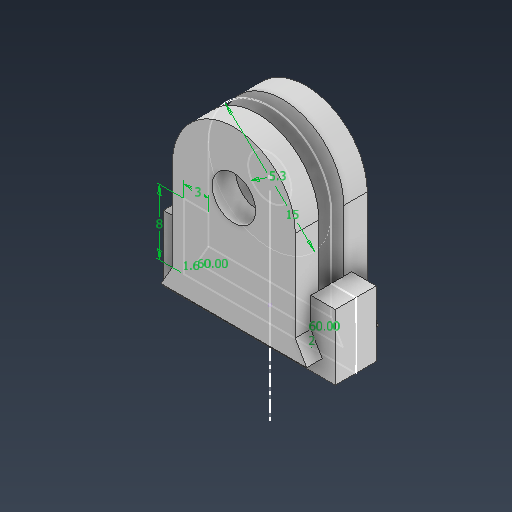
# Autodesk Inventor part: base
Saved by Autodesk Inventor 2025.3 (Build 293356000, 356)
## iProperties
Created: 2025-11-24
Part Number: base
Material: 一般
Document SubType Name: Modeling
Designer: 陳泓任
Density: 1 g/cm^3
Appearance: 預設
Author: 陳泓任
Autodesk Inventor part; units mm, degrees
ref_plane "YZ Plane" through (0, 0, 0) normal (1, 0, 0) x (0, 1, 0)
ref_plane "XZ Plane" through (0, 0, 0) normal (0, 1, 0) x (-1, 0, 0)
ref_plane "XY Plane" through (0, 0, 0) normal (0, 0, 1) x (1, 0, 0)
sketch "草圖1" plane through (0, 0, 0) normal (0, 0, 1) x (1, 0, 0)
  line L0 (0, 14.1483) -> (0, -10.3645)
  line L1 (0, 0) -> (-10.5, 0)
  line L2 (-10.5, 0) -> (-10.5, 8)
  line L3 (-10.5, 8) -> (-7.5, 8)
  line L4 (0, 0) -> (10.5, 0)
  line L5 (10.5, 0) -> (10.5, 8)
  line L6 (10.5, 8) -> (7.5, 8)
  circle A0 centre (0, 15.5) radius 2.65
  circle A1 centre (0, 15.5) radius 7.5 construction
  line L7 (-7.5, 4.4249) -> (-8.9, 2)
  line L8 (-8.9, 2) -> (0.3304, 2)
  line L9 (0.3304, 2) -> (8.9, 2)
  line L10 (8.9, 2) -> (7.5, 4.4249)
  line L11 (7.5, 4.4249) -> (7.5, 8.209)
  line L12 (-7.5, 8.147) -> (-7.5, 4.4249)
  line L13 (-7.5, 8.147) -> (-7.5, 15.5)
  line L14 (7.5, 8.209) -> (7.5, 15.5)
  arc A2 (7.5, 15.5) -> (-7.5, 15.5) centre (0, 15.5) ccw
  line L15 (-7.5, 4.4249) -> (7.5, 4.4249)
  point P0 (0, 2)
  dimension "d4" = 8
  dimension "d5" = 3
  dimension "d7" = 5.3
  dimension "d14" = 15
  dimension "d19" = 60
  dimension "d20" = 1.6
  dimension "d21" = 2
  dimension "d22" = 60
  constraints: 32 end point, 5 vertical, 4 horizontal, 4 point on circle, 4 tangent, 3 centre point, 3 point on line, 3 symmetric about line, 2 collinear, 1 coincident, 1 concentric, 1 perpendicular
  measures "d4" distance of L1.end L2.end
  measures "d5" distance of L2.end L3.end
  measures "d7" diameter of A0
  measures "d14" diameter of A1
  measures "d19" angle of L8 L7
  measures "d20" distance from line of L2 L7.end
  measures "d21" distance between parallel lines of L4 L9
  measures "d22" angle of L9 L10
extrude "擠出1" add sketch "草圖1" along normal mid plane 5 contours L8 L9 L10 L11 L6 L5 L4 L0 | L0 L1 L2 L3 L12 L7 L8
extrude "擠出2" add sketch "草圖1" along normal mid plane 8.8 separate body contours L15 L10 L9 L8 L0 | L0 L8 L7 L15 | L15 L12 L13 A2 L14 L11
extrude "擠出3" cut sketch "草圖1" along normal mid plane 3.05 contours L15 L12 L13 A2 L14 L11 bodies 2
